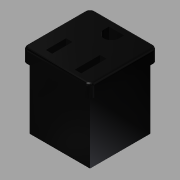
# Autodesk Inventor part: 739W-X203
Saved by Autodesk Inventor 2013 (Build 170138000, 138)
## iProperties
Created: 2014-06-07
Part Number: 739W-X203
Material: Generic
Document SubType Name: Modeling
Designer: Brad
Density: 1 g/cm^3
Author: Brad
Autodesk Inventor part; units mm, degrees
ref_plane "YZ Plane" through (0, 0, 0) normal (1, 0, 0) x (0, 1, 0)
ref_plane "XZ Plane" through (0, 0, 0) normal (0, 1, 0) x (-1, 0, 0)
ref_plane "XY Plane" through (0, 0, 0) normal (0, 0, 1) x (1, 0, 0)
sketch "Sketch1" plane through (0, 0, 0) normal (0, 0, 1) x (1, 0, 0)
  line L0 (-13.5, 13.5) -> (13.5, 13.5)
  line L1 (13.5, 13.5) -> (13.5, -13.5)
  line L2 (13.5, -13.5) -> (-13.5, -13.5)
  line L3 (-13.5, -13.5) -> (-13.5, 13.5)
  point P0 (0, 0)
  dimension "d0" = 27
  dimension "d2" = 27
  dimension "d3" = 13.5
  dimension "d4" = 13.5
  constraints: 8 end point, 2 parallel, 1 horizontal, 1 perpendicular
  measures "d0" distance of L0.end L1.end
  measures "d2" distance of L0.start L0.end
  measures "d3" distance from line of point (0, 0) L1
  measures "d4" distance from line of point (0, 0) L2
extrude "Extrusion1" add sketch "Sketch1" against normal blind 5
sketch "Sketch2" plane through (0, 0, -5) normal (0, 0, -1) x (-1, 0, 0)
  line L0 (13.5, 13.5) -> (-13.5, 13.5) projected
  line L1 (-13.5, 13.5) -> (-13.5, -13.5) projected
  line L2 (-12, 12) -> (12, 12)
  line L3 (12, 12) -> (12, -12)
  line L4 (12, -12) -> (-12, -12)
  line L5 (-12, -12) -> (-12, 12)
  point P0 (0, 0)
  dimension "d7" = 24
  dimension "d8" = 24
  dimension "d9" = 1.5
  dimension "d10" = 1.5
  constraints: 8 end point, 2 parallel, 1 horizontal, 1 perpendicular
  measures "d7" distance of L3.end L4.end
  measures "d8" distance of L2.end L3.end
  measures "d9" distance between parallel lines of L0 L2
  measures "d10" distance between parallel lines of L1 L5
extrude "Extrusion2" add sketch "Sketch2" along normal blind 25
sketch "Sketch3" plane through (0, 0, 0) normal (0, 0, 1) x (1, 0, 0)
  line L0 (-13.5, 13.5) -> (13.5, 13.5) projected
  line L1 (13.5, 13.5) -> (13.5, -13.5) projected
  line L2 (-3, 10.5) -> (3, 10.5)
  line L3 (3, 10.5) -> (3, 8.5)
  line L4 (-3, 10.5) -> (-3, 8.5)
  arc A0 (-3, 8.5) -> (3, 8.5) centre (0, 8.5) ccw
  line L5 (-7.5, -2) -> (-5, -2)
  line L6 (-5, -2) -> (-5, -10)
  line L7 (-5, -10) -> (-7.5, -10)
  line L8 (-7.5, -10) -> (-7.5, -2)
  line L9 (5, -1) -> (7.5, -1)
  line L10 (7.5, -1) -> (7.5, -11)
  line L11 (7.5, -11) -> (5, -11)
  line L12 (5, -11) -> (5, -1)
  point P0 (0, 0)
  dimension "d13" = 6
  dimension "d15" = 2
  dimension "d18" = 0
  dimension "d19" = 3
  dimension "d20" = 2.5
  dimension "d21" = 2.5
  dimension "d22" = 10
  dimension "d23" = 8
  dimension "d24" = 5
  dimension "d25" = 5
  dimension "d26" = 1
  dimension "d27" = 2
  constraints: 22 end point, 5 parallel, 4 perpendicular, 2 horizontal, 2 point on circle, 2 tangent, 1 centre point
  measures "d13" distance of L2.start L2.end
  measures "d15" distance of L4.end L2.start
  measures "d18" horizontal distance of point (0, 0) A0.centre
  measures "d19" distance between parallel lines of L0 L2
  measures "d20" distance of L5.start L5.end
  measures "d21" distance of L9.start L9.end
  measures "d22" distance of L9.end L10.end
  measures "d23" distance of L5.end L6.end
  measures "d24" distance from line of point (0, 0) L6
  measures "d25" distance from line of point (0, 0) L12
  measures "d26" distance from line of point (0, 0) L9
  measures "d27" distance from line of point (0, 0) L5
extrude "Extrusion3" cut sketch "Sketch3" against normal blind 20
fillet "Fillet1" radius 2 4 edges at (13.5, 13.5, -2.5) (13.5, -13.5, -2.5) (-13.5, -13.5, -2.5) (-13.5, 13.5, -2.5)
fillet "Fillet2" radius 1 8 edges at (12.9142, -12.9142, 0) (0, -13.5, 0) (-12.9142, -12.9142, 0) (-13.5, 0, 0) (-12.9142, 12.9142, 0) (0, 13.5, 0) (12.9142, 12.9142, 0) (13.5, 0, 0)
body "Solid1"
